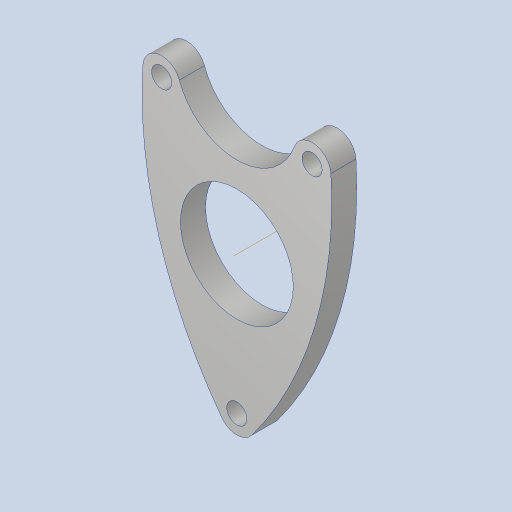
# Autodesk Inventor part: GP5-027
Saved by Autodesk Inventor 2023.4 (Build 274418000, 418)
## iProperties
Created: 2025-02-07
Part Number: GP5-027
Material: Aluminum 6061
Document SubType Name: Modeling
Designer: mavericks
Density: 2.7 g/cm^3
Appearance: Aluminum - Flat
Author: mavericks
Autodesk Inventor part; units mm, degrees
ref_plane "YZ Plane" through (0, 0, 0) normal (1, 0, 0) x (0, 1, 0)
ref_plane "XZ Plane" through (0, 0, 0) normal (0, 1, 0) x (-1, 0, 0)
ref_plane "XY Plane" through (0, 0, 0) normal (0, 0, 1) x (1, 0, 0)
sketch "Sketch1" plane through (0, 0, 0) normal (0, 0, 1) x (1, 0, 0)
  circle A0 centre (0, 0) radius 14.2875
  circle A1 centre (0, 0) radius 20.6375
  circle A2 centre (0, -34.925) radius 4.7625
  circle A3 centre (-19.05, 29.2721) radius 4.7625
  circle A4 centre (19.05, 29.2721) radius 4.7625
  arc A5 (-23.8032, 29.5703) -> (-3.8211, -37.7676) centre (78.1007, 23.1758) ccw
  arc A6 (3.8211, -37.7676) -> (23.8032, 29.5703) centre (-78.1007, 23.1758) ccw
  arc A7 (-14.5681, 30.8826) -> (14.5681, 30.8826) centre (0, 36.1176) ccw
  dimension "d0" = 28.575
  dimension "d1" = 6.35
  dimension "d2" = 9.525
  dimension "d3" = 9.525
  dimension "d4" = 9.525
  dimension "d7" = 9.525
  dimension "d8" = 9.525
  dimension "d9" = 9.525
  dimension "d13" = 19.05
  constraints: 12 point on circle, 9 tangent, 8 centre point, 5 coincident, 1 horizontal alignment, 1 vertical alignment
  measures "d0" diameter of A0
  measures "d1" radial gap between concentric circles of A0 A1
  measures "d2" diameter of A2
  measures "d3" diameter of A3
  measures "d4" diameter of A4
  measures "d13" horizontal distance of point (19.05, 29.272) point (0, 0)
extrude "Extrusion1" add sketch "Sketch1" against normal blind 6.35
hole "Hole1" at (0, 0, 0) at (-19.05, 29.2721, 0) at (19.05, 29.2721, 0) at (0, -34.925, 0) direction (0, 0, -1) diameter 5.1054 end through all clearance for "Flat Head Machine Screw (82)" size "#10" standard "Ansi Unified Screw Threads"
body "Solid1"
